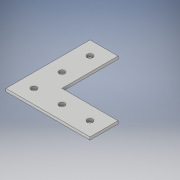
# Autodesk Inventor part: Bracing 3x3
Saved by Autodesk Inventor 2018 (Build 220112000, 112)
## iProperties
Created: 2019-01-19
Part Number: Bracing 3x3
Material: Generic
Document SubType Name: Modeling
Designer: Burni
Density: 1 g/cm^3
Appearance: Default
Author: Burni
Autodesk Inventor part; units mm, degrees
ref_plane "YZ Plane" through (0, 0, 0) normal (1, 0, 0) x (0, 1, 0)
ref_plane "XZ Plane" through (0, 0, 0) normal (0, 1, 0) x (-1, 0, 0)
ref_plane "XY Plane" through (0, 0, 0) normal (0, 0, 1) x (1, 0, 0)
sketch "Sketch1" plane through (0, 0, 0) normal (0, 1, 0) x (-1, 0, 0)
  line L0 (0, 0) -> (-25.4, 0)
  line L1 (-25.4, 0) -> (-25.4, 76.2)
  line L2 (-25.4, 76.2) -> (0, 76.2)
  line L3 (0, 76.2) -> (0, 0)
  line L4 (-25.4, 76.2) -> (-76.2, 76.2)
  line L5 (-76.2, 76.2) -> (-76.2, 50.8)
  line L6 (-76.2, 50.8) -> (-25.4, 50.8)
  line L7 (-25.4, 50.8) -> (-25.4, 76.2)
  circle A0 centre (-63.5, 63.5) radius 2.5797
  circle A1 centre (-38.1, 63.5) radius 2.5797
  circle A2 centre (-12.7, 63.5) radius 2.5797
  circle A3 centre (-12.7, 38.1) radius 2.5797
  circle A4 centre (-12.7, 12.7) radius 2.5797
  dimension "d0" = 0
  dimension "d1" = 25.4
  dimension "d2" = 76.2
  dimension "d3" = 50.8
  dimension "d4" = 25.4
  dimension "d5" = 12.7
  dimension "d6" = 12.7
  dimension "d7" = 12.7
  dimension "d8" = 12.7
  dimension "d9" = 25.4
  dimension "d10" = 25.4
  dimension "d11" = 5.1594
  dimension "d12" = 5.1594
  dimension "d13" = 5.1594
  dimension "d14" = 5.1594
  dimension "d15" = 5.1594
  dimension "d16" = 12.7
  dimension "d17" = 12.7
  dimension "d18" = 12.7
  dimension "d19" = 25.4
  dimension "d20" = 12.7
  constraints: 16 end point, 5 centre point, 4 parallel, 2 horizontal, 2 perpendicular, 1 point on line
  measures "d0" distance between parallel lines of L2 L4
  measures "d1" distance of L4.end L5.end
  measures "d2" distance of L2.end L0.start
  measures "d3" distance of L4.start L4.end
  measures "d4" distance of L1.end L2.end
  measures "d5" distance from line of L1 A4.centre
  measures "d6" distance from line of L1 A3.centre
  measures "d7" distance from line of L7 A2.centre
  measures "d8" distance from line of L2 A2.centre
  measures "d9" distance of A3.centre A2.centre
  measures "d10" distance of A3.centre A4.centre
  measures "d11" diameter of A3
  measures "d12" diameter of A4
  measures "d13" diameter of A2
  measures "d14" diameter of A1
  measures "d15" diameter of A0
  measures "d16" distance from line of L4 A1.centre
  measures "d17" distance from line of L4 A0.centre
  measures "d18" distance from line of A0.centre L5
  measures "d19" distance of A0.centre A1.centre
  measures "d20" distance from line of L1 A1.centre
extrude "Extrusion1" add sketch "Sketch1" along normal blind 2.54
equation "\"d6\" = d5"
equation "\"d7\" = d5"
equation "\"d12\" = d11"
equation "\"d13\" = d11"
equation "\"d14\" = d11"
equation "\"d15\" = d11"
body "Solid1"
